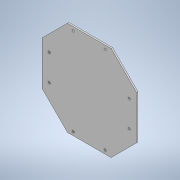
# Autodesk Inventor part: t960_power_distribution_board_TL2996
Saved by Autodesk Inventor 2020.2 (Build 242310000, 310)
## iProperties
Created: 2020-08-20
Part Number: t960_power_distribution_board_TL2996
Material: Generic
Document SubType Name: Modeling
Designer: Krishna Makhija
Density: 1 g/cm^3
Appearance: Default
Author: Krishna Makhija
Autodesk Inventor part; units mm, degrees
ref_plane "YZ Plane" through (0, 0, 0) normal (1, 0, 0) x (0, 1, 0)
ref_plane "XZ Plane" through (0, 0, 0) normal (0, 1, 0) x (-1, 0, 0)
ref_plane "XY Plane" through (0, 0, 0) normal (0, 0, 1) x (1, 0, 0)
sketch "Sketch1" plane through (0, 0, 0) normal (0, 0, 1) x (1, 0, 0)
  line L0 (-65.0002, 64.9999) -> (65.0002, 64.9999)
  line L1 (65.0002, 64.9999) -> (65.0002, -64.9999)
  line L2 (65.0002, -64.9999) -> (-65.0002, -64.9999)
  line L3 (-65.0002, -64.9999) -> (-65.0002, 64.9999)
  line L4 (-65.0002, 64.9999) -> (65.0002, -64.9999) construction
  line L5 (65.0002, 64.9999) -> (-65.0002, -64.9999) construction
  line L6 (30, -64.9999) -> (65.0002, -29.9994)
  line L7 (-29.9996, -64.9999) -> (-65.0002, -29.9995)
  line L8 (-29.9996, 64.9999) -> (-65.0002, 29.9995)
  line L9 (29.9986, 64.9999) -> (65.0002, 29.9981)
  point P0 (0, 0)
  constraints: 20 end point, 8 point on line, 4 perpendicular, 2 midpoint, 2 parallel, 1 horizontal
extrude "Extrusion1" add sketch "Sketch1" along normal blind 2 contours L0 L9 L1 L6 L2 L7 L3 L8
sketch "Sketch2" plane through (0, 0, 2) normal (0, 0, 1) x (1, 0, 0)
  circle A0 centre (22, 60) radius 1.4999
  circle A1 centre (-22, 60) radius 1.4999
  circle A2 centre (22, -60) radius 1.4999
  circle A3 centre (-22, -60) radius 1.4999
  circle A4 centre (55, 18) radius 1.4999
  circle A5 centre (55, -18) radius 1.4999
  circle A6 centre (-55, 18) radius 1.4999
  circle A7 centre (-54.9426, 18) radius 1.4999
  circle A8 centre (-55, -18) radius 1.4999
  circle A9 centre (-54.9426, -18) radius 1.4999
  point P0 (-54.9713, 16.5004)
  point P1 (-54.9713, 19.4996)
  point P2 (-54.9713, -19.4996)
  point P3 (-54.9713, -16.5004)
  constraints: 10 centre point
extrude "Extrusion2" cut sketch "Sketch2" against normal blind 10
body "Solid1"
